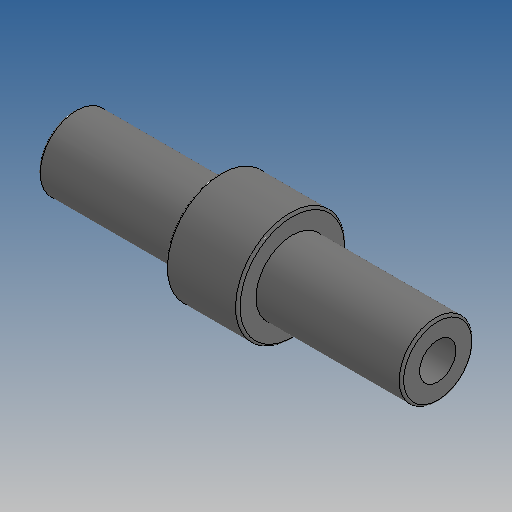
# Autodesk Inventor part: 78258-DarkStoneGrey
Saved by Autodesk Inventor 2025 (Build 290162010, 162A)
## iProperties
Created: 2021-12-28
Part Number: 78258-DarkStoneGrey
Material: ABS Plastic
Document SubType Name: Modeling
Designer: MARTIN CSANAKI
Density: 1.06 g/cm^3
Appearance: DkBluishGray
Mass: 0.153337 g
Surface Area: 2.51163 cm^2
Volume: 0.144658 cm^3
Author: MARTIN CSANAKI
Autodesk Inventor part; units mm, degrees
ref_plane "YZ Plane" through (0, 0, 0) normal (1, 0, 0) x (0, 1, 0)
ref_plane "XZ Plane" through (0, 0, 0) normal (0, 1, 0) x (-1, 0, 0)
ref_plane "XY Plane" through (0, 0, 0) normal (0, 0, 1) x (1, 0, 0)
sketch "Sketch1" plane through (0, 0, 0) normal (0, 0, 1) x (1, 0, 0)
  line L0 (0, 0) -> (-8, 0)
  line L1 (0, 2.4) -> (-1.6, 2.4)
  line L2 (-1.6, 2.4) -> (-1.6, 1.6)
  line L3 (-1.6, 1.6) -> (-8, 1.6)
  line L4 (-8, 1.6) -> (-8, 0.8)
  line L5 (-8, 0.8) -> (-4, 0.8)
  line L6 (-4, 0.8) -> (-4, 0)
  line L7 (0, 2.4) -> (0, 0) construction
  line L8 (0, 2.4) -> (1.6, 2.4)
  line L9 (1.6, 2.4) -> (1.6, 1.6)
  line L10 (1.6, 1.6) -> (8, 1.6)
  line L11 (8, 1.6) -> (8, 0.8)
  line L12 (8, 0.8) -> (4, 0.8)
  line L13 (4, 0.8) -> (4, 0)
  line L14 (-4, 0) -> (4, 0)
  dimension "d0" = 8
  dimension "d2" = 4.8
  dimension "d3" = 3.2
  dimension "d4" = 1.6
  dimension "d5" = 4
  dimension "d6" = 3.2
  constraints: 30 end point, 6 symmetric about line, 5 perpendicular, 3 horizontal, 1 midpoint, 1 parallel, 1 vertical alignment
  measures "d0" distance of L0.start L0.end
  measures "d2" diameter of L1 L0
  measures "d3" diameter of L3 L0
  measures "d4" diameter of L5 L0
  measures "d5" distance of L4.end L5.end
  measures "d6" distance between parallel lines of L9 L2
revolve "Revolution1" add sketch "Sketch1" angle 360 about axis through (0, 0, 0) along (-1, 0, 0)
fillet "Fillet1" radius 0.1 4 edges at (-1.6, -2.4, 0) (1.6, -2.4, 0) (8, -1.6, 0) (-8, -1.6, 0)
equation "\"d0\" = lu"
equation "\"d2\" = kd"
equation "\"d3\" = rd"
equation "\"d4\" = 0.5 * rd"
equation "\"d5\" = 0.5 * lu"
equation "\"d6\" = rd"
equation "\"d8\" = lf"
equation "\"lu\" = 8"
equation "\"kd\" = 4.8"
equation "\"rd\" = 3.2"
equation "\"lf\" = 0.1"
body "Solid1"
